Post Sign (Autodesk Fusion 360 design; units mm, degrees)
Autodesk Fusion 360 part; units mm, degrees
(part 1 of 5)
sketch "Sketch1" plane through (0, 0, 0) normal (0, 0, 1) x (1, 0, 0)
  spline S0 degree 3 poles (15.8654, 98.7935) (15.4934, 98.9562) (15.1331, 99.0376) (14.7843, 99.0376) knots 0 0 0 0 1 1 1 1
  spline S1 degree 3 poles (14.7843, 99.0376) (14.4356, 99.0376) (14.0868, 98.8167) (13.7381, 98.375) knots 0 0 0 0 1 1 1 1
  spline S2 degree 3 poles (13.7381, 98.375) (13.3894, 97.9332) (13.1568, 97.2939) (13.0406, 96.4569) knots 0 0 0 0 1 1 1 1
  line L0 (13.0406, 96.4569) -> (11.2969, 84.2509)
  spline S3 degree 3 poles (11.2969, 84.2509) (14.2263, 85.5296) (16.0979, 86.4829) (16.9117, 87.1106) knots 0 0 0 0 1 1 1 1
  line L1 (16.9117, 87.1106) -> (18.2369, 84.8089)
  spline S4 degree 3 poles (18.2369, 84.8089) (17.5394, 84.2742) (16.7024, 83.7975) (15.7259, 83.3791) knots 0 0 0 0 1 1 1 1
  spline S5 degree 3 poles (15.7259, 83.3791) (14.7495, 82.9606) (13.8078, 82.5653) (12.9011, 82.1933) knots 0 0 0 0 1 1 1 1
  spline S6 degree 3 poles (12.9011, 82.1933) (11.9944, 81.8446) (11.3202, 81.5772) (10.8784, 81.3912) knots 0 0 0 0 1 1 1 1
  line L2 (10.8784, 81.3912) -> (9.7276, 73.2307)
  spline S7 degree 3 poles (9.7276, 73.2307) (9.4253, 70.9987) (8.6232, 69.3596) (7.3212, 68.3134) knots 0 0 0 0 1 1 1 1
  spline S8 degree 3 poles (7.3212, 68.3134) (6.0425, 67.2439) (4.6243, 66.7092) (3.0666, 66.7092) knots 0 0 0 0 1 1 1 1
  spline S9 degree 3 poles (3.0666, 66.7092) (1.5321, 66.7092) (0.3115, 67.2788) (-0.5952, 68.418) knots 0 0 0 0 1 1 1 1
  spline S10 degree 3 poles (-0.5952, 68.418) (-1.5019, 69.534) (-1.9553, 70.7895) (-1.9553, 72.1844) knots 0 0 0 0 1 1 1 1
  spline S11 degree 3 poles (-1.9553, 72.1844) (-1.9553, 75.8346) (0.7184, 79.0779) (6.0658, 81.9143) knots 0 0 0 0 1 1 1 1
  line L3 (6.0658, 81.9143) -> (6.4145, 84.7391)
  spline S12 degree 3 poles (6.4145, 84.7391) (6.8563, 88.7381) (7.3096, 92.2138) (7.7746, 95.1665) knots 0 0 0 0 1 1 1 1
  spline S13 degree 3 poles (7.7746, 95.1665) (6.4494, 94.6318) (5.0544, 94.3644) (3.5897, 94.3644) knots 0 0 0 0 1 1 1 1
  spline S14 degree 3 poles (3.5897, 94.3644) (2.1482, 94.3644) (0.9741, 94.7597) (0.0674, 95.5502) knots 0 0 0 0 1 1 1 1
  spline S15 degree 3 poles (0.0674, 95.5502) (-0.8161, 96.3407) (-1.2578, 97.3752) (-1.2578, 98.654) knots 0 0 0 0 1 1 1 1
  spline S16 degree 3 poles (-1.2578, 98.654) (-1.2578, 99.9327) (-0.8044, 100.9324) (0.1023, 101.6531) knots 0 0 0 0 1 1 1 1
  spline S17 degree 3 poles (0.1023, 101.6531) (1.0323, 102.3971) (2.1947, 102.7691) (3.5897, 102.7691) knots 0 0 0 0 1 1 1 1
  spline S18 degree 3 poles (3.5897, 102.7691) (4.45, 102.7691) (5.6822, 102.5017) (7.2864, 101.967) knots 0 0 0 0 1 1 1 1
  spline S19 degree 3 poles (7.2864, 101.967) (8.9139, 101.4323) (10.1693, 101.1649) (11.0528, 101.1649) knots 0 0 0 0 1 1 1 1
  spline S20 degree 3 poles (11.0528, 101.1649) (12.6337, 101.1649) (13.959, 101.5718) (15.0284, 102.3855) knots 0 0 0 0 1 1 1 1
  spline S21 degree 3 poles (15.0284, 102.3855) (15.6097, 101.5718) (15.9003, 100.6069) (15.9003, 99.4909) knots 0 0 0 0 1 1 1 1
  spline S22 degree 3 poles (15.9003, 99.4909) (15.9003, 99.2584) (15.8887, 99.026) (15.8654, 98.7935) knots 0 0 0 0 1 1 1 1
  spline S23 degree 3 poles (2.1947, 97.7124) (2.1947, 97.3636) (2.3807, 97.0614) (2.7527, 96.8056) knots 0 0 0 0 1 1 1 1
  spline S24 degree 3 poles (2.7527, 96.8056) (3.1479, 96.5499) (3.7292, 96.422) (4.4964, 96.422) knots 0 0 0 0 1 1 1 1
  spline S25 degree 3 poles (4.4964, 96.422) (5.2869, 96.422) (6.3099, 96.7707) (7.5654, 97.4682) knots 0 0 0 0 1 1 1 1
  spline S26 degree 3 poles (7.5654, 97.4682) (6.6586, 97.6775) (5.7286, 97.91) (4.7754, 98.1657) knots 0 0 0 0 1 1 1 1
  spline S27 degree 3 poles (4.7754, 98.1657) (3.8222, 98.4447) (3.2526, 98.5842) (3.0666, 98.5842) knots 0 0 0 0 1 1 1 1
  spline S28 degree 3 poles (3.0666, 98.5842) (2.4854, 98.5842) (2.1947, 98.2936) (2.1947, 97.7124) knots 0 0 0 0 1 1 1 1
  spline S29 degree 3 poles (5.6822, 78.8803) (2.3575, 76.8808) (0.6951, 74.7651) (0.6951, 72.5332) knots 0 0 0 0 1 1 1 1
  spline S30 degree 3 poles (0.6951, 72.5332) (0.6951, 71.9054) (0.8579, 71.3707) (1.1834, 70.929) knots 0 0 0 0 1 1 1 1
  spline S31 degree 3 poles (1.1834, 70.929) (1.5554, 70.4175) (2.0204, 70.1617) (2.5784, 70.1617) knots 0 0 0 0 1 1 1 1
  spline S32 degree 3 poles (2.5784, 70.1617) (3.1596, 70.1617) (3.6595, 70.3361) (4.0779, 70.6848) knots 0 0 0 0 1 1 1 1
  spline S33 degree 3 poles (4.0779, 70.6848) (4.4964, 71.0336) (4.7522, 71.5916) (4.8452, 72.3588) knots 0 0 0 0 1 1 1 1
  line L4 (4.8452, 72.3588) -> (5.6822, 78.8803)
  spline S34 degree 3 poles (29.2909, 92.6905) (28.3377, 85.1576) (27.8611, 81.1471) (27.8611, 80.6589) knots 0 0 0 0 1 1 1 1
  spline S35 degree 3 poles (27.8611, 80.6589) (27.8611, 79.7289) (28.1982, 79.2639) (28.8724, 79.2639) knots 0 0 0 0 1 1 1 1
  spline S36 degree 3 poles (28.8724, 79.2639) (29.4769, 79.2639) (30.1279, 79.6708) (30.8254, 80.4845) knots 0 0 0 0 1 1 1 1
  spline S37 degree 3 poles (30.8254, 80.4845) (31.5461, 81.3215) (32.1157, 82.5653) (32.5342, 84.216) knots 0 0 0 0 1 1 1 1
  spline S38 degree 3 poles (32.5342, 84.216) (33.3014, 83.3791) (33.7664, 82.728) (33.9292, 82.2631) knots 0 0 0 0 1 1 1 1
  spline S39 degree 3 poles (33.9292, 82.2631) (33.3945, 80.0079) (32.5458, 78.4153) (31.3834, 77.4853) knots 0 0 0 0 1 1 1 1
  spline S40 degree 3 poles (31.3834, 77.4853) (30.2209, 76.5553) (29.0235, 76.0903) (27.7913, 76.0903) knots 0 0 0 0 1 1 1 1
  spline S41 degree 3 poles (27.7913, 76.0903) (25.7686, 76.0903) (24.4085, 76.8692) (23.711, 78.4269) knots 0 0 0 0 1 1 1 1
  spline S42 degree 3 poles (23.711, 78.4269) (22.502, 76.8692) (20.8862, 76.0903) (18.8635, 76.0903) knots 0 0 0 0 1 1 1 1
  spline S43 degree 3 poles (18.8635, 76.0903) (17.1896, 76.0903) (15.8992, 76.5088) (14.9925, 77.3458) knots 0 0 0 0 1 1 1 1
  spline S44 degree 3 poles (14.9925, 77.3458) (14.0857, 78.1828) (13.6324, 79.2755) (13.6324, 80.624) knots 0 0 0 0 1 1 1 1
  spline S45 degree 3 poles (13.6324, 80.624) (13.6324, 80.9495) (13.6905, 81.5191) (13.8068, 82.3328) knots 0 0 0 0 1 1 1 1
  spline S46 degree 3 poles (13.8068, 82.3328) (14.3415, 86.6572) (14.7484, 90.0982) (15.0274, 92.6556) knots 0 0 0 0 1 1 1 1
  spline S47 degree 3 poles (15.0274, 92.6556) (15.7481, 92.9113) (16.4107, 93.0392) (17.0152, 93.0392) knots 0 0 0 0 1 1 1 1
  spline S48 degree 3 poles (17.0152, 93.0392) (17.6197, 93.0392) (18.073, 93.0159) (18.3753, 92.9695) knots 0 0 0 0 1 1 1 1
  spline S49 degree 3 poles (18.3753, 92.9695) (18.6775, 92.923) (18.9681, 92.7486) (19.2471, 92.4463) knots 0 0 0 0 1 1 1 1
  spline S50 degree 3 poles (19.2471, 92.4463) (19.5261, 92.1441) (19.6656, 91.714) (19.6656, 91.156) knots 0 0 0 0 1 1 1 1
  line L5 (19.6656, 91.156) -> (18.5148, 82.2631)
  spline S51 degree 3 poles (18.5148, 82.2631) (18.4683, 81.9841) (18.445, 81.7284) (18.445, 81.4958) knots 0 0 0 0 1 1 1 1
  spline S52 degree 3 poles (18.445, 81.4958) (18.445, 80.1241) (19.0728, 79.4383) (20.3282, 79.4383) knots 0 0 0 0 1 1 1 1
  spline S53 degree 3 poles (20.3282, 79.4383) (21.4907, 79.4383) (22.4556, 80.0079) (23.2228, 81.1471) knots 0 0 0 0 1 1 1 1
  spline S54 degree 3 poles (23.2228, 81.1471) (23.2228, 81.4028) (23.2461, 81.8097) (23.2925, 82.3677) knots 0 0 0 0 1 1 1 1
  line L6 (23.2925, 82.3677) -> (24.4434, 91.6442)
  spline S55 degree 3 poles (24.4434, 91.6442) (24.6062, 92.0395) (24.9549, 92.365) (25.4896, 92.6207) knots 0 0 0 0 1 1 1 1
  spline S56 degree 3 poles (25.4896, 92.6207) (26.0243, 92.8997) (26.6869, 93.0392) (27.4774, 93.0392) knots 0 0 0 0 1 1 1 1
  spline S57 degree 3 poles (27.4774, 93.0392) (28.2912, 93.0392) (28.8957, 92.923) (29.2909, 92.6905) knots 0 0 0 0 1 1 1 1
  line L7 (40.9332, 80.2404) -> (41.7701, 87.9476)
  spline S58 degree 3 poles (41.7701, 87.9476) (41.7701, 88.5753) (41.6074, 89.0984) (41.2819, 89.5169) knots 0 0 0 0 1 1 1 1
  spline S59 degree 3 poles (41.2819, 89.5169) (40.9564, 89.9354) (40.4333, 90.1446) (39.7126, 90.1446) knots 0 0 0 0 1 1 1 1
  spline S60 degree 3 poles (39.7126, 90.1446) (38.9919, 90.1446) (38.3757, 89.854) (37.8642, 89.2728) knots 0 0 0 0 1 1 1 1
  spline S61 degree 3 poles (37.8642, 89.2728) (37.376, 88.7148) (37.0156, 87.9708) (36.7831, 87.0408) knots 0 0 0 0 1 1 1 1
  spline S62 degree 3 poles (36.7831, 87.0408) (36.6204, 85.7156) (36.3763, 83.7743) (36.0508, 81.2168) knots 0 0 0 0 1 1 1 1
  spline S63 degree 3 poles (36.0508, 81.2168) (35.7253, 78.6826) (35.5161, 77.0319) (35.423, 76.2647) knots 0 0 0 0 1 1 1 1
  line L8 (35.423, 76.2647) -> (30.7848, 76.2647)
  spline S64 degree 3 poles (30.7848, 76.2647) (32.4587, 90.5167) (33.4701, 99.2701) (33.8188, 102.525) knots 0 0 0 0 1 1 1 1
  spline S65 degree 3 poles (33.8188, 102.525) (34.3071, 102.711) (34.9697, 102.804) (35.8067, 102.804) knots 0 0 0 0 1 1 1 1
  spline S66 degree 3 poles (35.8067, 102.804) (37.6201, 102.804) (38.5268, 102.2693) (38.5268, 101.1998) knots 0 0 0 0 1 1 1 1
  line L9 (38.5268, 101.1998) -> (38.5268, 100.9905)
  spline S67 degree 3 poles (38.5268, 100.9905) (38.1316, 97.3403) (37.7131, 94.1319) (37.2714, 91.3652) knots 0 0 0 0 1 1 1 1
  spline S68 degree 3 poles (37.2714, 91.3652) (38.5036, 92.4812) (39.8986, 93.0392) (41.4563, 93.0392) knots 0 0 0 0 1 1 1 1
  spline S69 degree 3 poles (41.4563, 93.0392) (43.014, 93.0392) (44.2462, 92.644) (45.1529, 91.8535) knots 0 0 0 0 1 1 1 1
  spline S70 degree 3 poles (45.1529, 91.8535) (46.0597, 91.063) (46.513, 90.0633) (46.513, 88.8543) knots 0 0 0 0 1 1 1 1
  spline S71 degree 3 poles (46.513, 88.8543) (46.513, 88.5288) (46.4433, 87.9243) (46.3038, 87.0408) knots 0 0 0 0 1 1 1 1
  spline S72 degree 3 poles (46.3038, 87.0408) (45.7691, 83.5534) (45.5017, 81.5075) (45.5017, 80.903) knots 0 0 0 0 1 1 1 1
  spline S73 degree 3 poles (45.5017, 80.903) (45.5017, 79.8103) (45.8621, 79.2639) (46.5828, 79.2639) knots 0 0 0 0 1 1 1 1
  spline S74 degree 3 poles (46.5828, 79.2639) (47.1873, 79.2639) (47.8266, 79.6591) (48.5007, 80.4496) knots 0 0 0 0 1 1 1 1
  spline S75 degree 3 poles (48.5007, 80.4496) (49.1982, 81.2633) (49.7562, 82.5072) (50.1747, 84.1812) knots 0 0 0 0 1 1 1 1
  spline S76 degree 3 poles (50.1747, 84.1812) (50.9653, 83.3442) (51.4421, 82.6816) (51.6045, 82.1933) knots 0 0 0 0 1 1 1 1
  spline S77 degree 3 poles (51.6045, 82.1933) (50.3959, 78.1479) (48.2566, 76.1252) (45.1878, 76.1252) knots 0 0 0 0 1 1 1 1
  spline S78 degree 3 poles (45.1878, 76.1252) (43.7464, 76.1252) (42.6769, 76.567) (41.9794, 77.4504) knots 0 0 0 0 1 1 1 1
  spline S79 degree 3 poles (41.9794, 77.4504) (41.2819, 78.3339) (40.9332, 79.2639) (40.9332, 80.2404) knots 0 0 0 0 1 1 1 1
  spline S80 degree 3 poles (64.2664, 76.0903) (62.1276, 76.0903) (60.7092, 76.8343) (60.0117, 78.3223) knots 0 0 0 0 1 1 1 1
  spline S81 degree 3 poles (60.0117, 78.3223) (58.8031, 76.8111) (57.2452, 76.0555) (55.3386, 76.0555) knots 0 0 0 0 1 1 1 1
  spline S82 degree 3 poles (55.3386, 76.0555) (53.4553, 76.0555) (51.8631, 76.6948) (50.5608, 77.9735) knots 0 0 0 0 1 1 1 1
  spline S83 degree 3 poles (50.5608, 77.9735) (49.2824, 79.2523) (48.6427, 80.9379) (48.6427, 83.0303) knots 0 0 0 0 1 1 1 1
  spline S84 degree 3 poles (48.6427, 83.0303) (48.6427, 86.076) (49.538, 88.5056) (51.328, 90.319) knots 0 0 0 0 1 1 1 1
  spline S85 degree 3 poles (51.328, 90.319) (53.1186, 92.1325) (55.3854, 93.0392) (58.1285, 93.0392) knots 0 0 0 0 1 1 1 1
  spline S86 degree 3 poles (58.1285, 93.0392) (58.1982, 93.0392) (58.268, 93.0392) (58.3377, 93.0392) knots 0 0 0 0 1 1 1 1
  spline S87 degree 3 poles (58.3377, 93.0392) (59.5005, 93.0392) (60.5697, 92.8416) (61.5462, 92.4463) knots 0 0 0 0 1 1 1 1
  spline S88 degree 3 poles (61.5462, 92.4463) (62.1739, 92.8416) (62.9297, 93.0392) (63.813, 93.0392) knots 0 0 0 0 1 1 1 1
  spline S89 degree 3 poles (63.813, 93.0392) (64.7197, 93.0392) (65.3709, 92.923) (65.7659, 92.6905) knots 0 0 0 0 1 1 1 1
  spline S90 degree 3 poles (65.7659, 92.6905) (65.5567, 90.97) (65.336, 89.2728) (65.1033, 87.5988) knots 0 0 0 0 1 1 1 1
  spline S91 degree 3 poles (65.1033, 87.5988) (64.8712, 85.9481) (64.7083, 84.774) (64.6151, 84.0765) knots 0 0 0 0 1 1 1 1
  spline S92 degree 3 poles (64.6151, 84.0765) (64.4058, 82.4956) (64.3012, 81.3563) (64.3012, 80.6589) knots 0 0 0 0 1 1 1 1
  spline S93 degree 3 poles (64.3012, 80.6589) (64.3012, 79.7289) (64.6734, 79.2639) (65.4172, 79.2639) knots 0 0 0 0 1 1 1 1
  spline S94 degree 3 poles (65.4172, 79.2639) (65.9986, 79.2639) (66.6149, 79.6475) (67.2655, 80.4147) knots 0 0 0 0 1 1 1 1
  spline S95 degree 3 poles (67.2655, 80.4147) (67.9167, 81.2052) (68.4861, 82.4374) (68.9744, 84.1114) knots 0 0 0 0 1 1 1 1
  spline S96 degree 3 poles (68.9744, 84.1114) (69.6489, 83.5069) (70.1138, 82.8327) (70.3693, 82.0887) knots 0 0 0 0 1 1 1 1
  spline S97 degree 3 poles (70.3693, 82.0887) (69.6953, 79.88) (68.7885, 78.3223) (67.6492, 77.4156) knots 0 0 0 0 1 1 1 1
  spline S98 degree 3 poles (67.6492, 77.4156) (66.5103, 76.5321) (65.3823, 76.0903) (64.2664, 76.0903) knots 0 0 0 0 1 1 1 1
  spline S99 degree 3 poles (58.6516, 90.319) (57.164, 90.319) (55.9782, 89.7494) (55.0944, 88.6102) knots 0 0 0 0 1 1 1 1
  spline S100 degree 3 poles (55.0944, 88.6102) (54.2345, 87.4942) (53.7229, 85.8202) (53.56, 83.5883) knots 0 0 0 0 1 1 1 1
  spline S101 degree 3 poles (53.56, 83.5883) (53.5371, 83.3791) (53.5251, 83.1814) (53.5251, 82.9954) knots 0 0 0 0 1 1 1 1
  spline S102 degree 3 poles (53.5251, 82.9954) (53.5251, 81.8562) (53.7926, 80.9495) (54.3272, 80.2752) knots 0 0 0 0 1 1 1 1
  spline S103 degree 3 poles (54.3272, 80.2752) (54.8852, 79.601) (55.5946, 79.2639) (56.4545, 79.2639) knots 0 0 0 0 1 1 1 1
  spline S104 degree 3 poles (56.4545, 79.2639) (57.9192, 79.2639) (59.0238, 80.2985) (59.7676, 82.3677) knots 0 0 0 0 1 1 1 1
  line L10 (59.7676, 82.3677) -> (60.6046, 89.9005)
  spline S105 degree 3 poles (60.6046, 89.9005) (59.9305, 90.1795) (59.2793, 90.319) (58.6516, 90.319) knots 0 0 0 0 1 1 1 1
  spline S106 degree 3 poles (82.4308, 86.9362) (84.2677, 85.5877) (85.1859, 83.9952) (85.1859, 82.1585) knots 0 0 0 0 1 1 1 1
  spline S107 degree 3 poles (85.1859, 82.1585) (85.1859, 80.3217) (84.465, 78.8454) (83.0237, 77.7294) knots 0 0 0 0 1 1 1 1
  spline S108 degree 3 poles (83.0237, 77.7294) (81.5824, 76.6135) (79.7689, 76.0555) (77.5833, 76.0555) knots 0 0 0 0 1 1 1 1
  spline S109 degree 3 poles (77.5833, 76.0555) (76.1649, 76.0555) (74.9792, 76.4042) (74.0261, 77.1017) knots 0 0 0 0 1 1 1 1
  spline S110 degree 3 poles (74.0261, 77.1017) (73.096, 77.8224) (72.6312, 78.7059) (72.6312, 79.7521) knots 0 0 0 0 1 1 1 1
  spline S111 degree 3 poles (72.6312, 79.7521) (72.6312, 80.7984) (72.9799, 81.6237) (73.6774, 82.2282) knots 0 0 0 0 1 1 1 1
  spline S112 degree 3 poles (73.6774, 82.2282) (74.3749, 82.8559) (75.2468, 83.2396) (76.293, 83.3791) knots 0 0 0 0 1 1 1 1
  spline S113 degree 3 poles (76.293, 83.3791) (75.8047, 82.6816) (75.5606, 82.0073) (75.5606, 81.3563) knots 0 0 0 0 1 1 1 1
  spline S114 degree 3 poles (75.5606, 81.3563) (75.5606, 80.7286) (75.7813, 80.2171) (76.2232, 79.8219) knots 0 0 0 0 1 1 1 1
  spline S115 degree 3 poles (76.2232, 79.8219) (76.6651, 79.4267) (77.2231, 79.229) (77.8972, 79.229) knots 0 0 0 0 1 1 1 1
  spline S116 degree 3 poles (77.8972, 79.229) (78.5713, 79.229) (79.1292, 79.4731) (79.5712, 79.9614) knots 0 0 0 0 1 1 1 1
  spline S117 degree 3 poles (79.5712, 79.9614) (80.0131, 80.4729) (80.2338, 81.0541) (80.2338, 81.7051) knots 0 0 0 0 1 1 1 1
  spline S118 degree 3 poles (80.2338, 81.7051) (80.2338, 82.7746) (79.7341, 83.7278) (78.7342, 84.5648) knots 0 0 0 0 1 1 1 1
  spline S119 degree 3 poles (78.7342, 84.5648) (78.1298, 85.053) (77.4787, 85.5064) (76.7812, 85.9249) knots 0 0 0 0 1 1 1 1
  spline S120 degree 3 poles (76.7812, 85.9249) (76.0837, 86.3666) (75.7116, 86.5991) (75.6652, 86.6224) knots 0 0 0 0 1 1 1 1
  spline S121 degree 3 poles (75.6652, 86.6224) (75.5721, 86.6921) (75.4794, 86.7502) (75.3862, 86.7967) knots 0 0 0 0 1 1 1 1
  spline S122 degree 3 poles (75.3862, 86.7967) (74.9678, 86.3085) (74.3634, 85.6343) (73.5728, 84.774) knots 0 0 0 0 1 1 1 1
  spline S123 degree 3 poles (73.5728, 84.774) (72.7821, 83.937) (72.1544, 83.2628) (71.6896, 82.7513) knots 0 0 0 0 1 1 1 1
  spline S124 degree 3 poles (71.6896, 82.7513) (70.3878, 81.3331) (69.6554, 80.1474) (69.4925, 79.1941) knots 0 0 0 0 1 1 1 1
  spline S125 degree 3 poles (69.4925, 79.1941) (69.4462, 79.0082) (69.4228, 78.6478) (69.4228, 78.113) knots 0 0 0 0 1 1 1 1
  spline S126 degree 3 poles (69.4228, 78.113) (69.4228, 77.6015) (69.5737, 77.0668) (69.8761, 76.5088) knots 0 0 0 0 1 1 1 1
  spline S127 degree 3 poles (69.8761, 76.5088) (70.2015, 75.9508) (70.5851, 75.5324) (71.027, 75.2534) knots 0 0 0 0 1 1 1 1
  spline S128 degree 3 poles (71.027, 75.2534) (71.4689, 74.9744) (71.8988, 74.7535) (72.3173, 74.5907) knots 0 0 0 0 1 1 1 1
  spline S129 degree 3 poles (72.3173, 74.5907) (72.7592, 74.4048) (73.1309, 74.2769) (73.4333, 74.2071) knots 0 0 0 0 1 1 1 1
  spline S130 degree 3 poles (73.4333, 74.2071) (73.7586, 74.1374) (73.9215, 74.0909) (73.9215, 74.0676) knots 0 0 0 0 1 1 1 1
  spline S131 degree 3 poles (73.9215, 74.0676) (73.9215, 73.9049) (73.666, 73.7189) (73.1543, 73.5096) knots 0 0 0 0 1 1 1 1
  spline S132 degree 3 poles (73.1543, 73.5096) (72.2012, 73.1609) (71.2013, 72.9865) (70.1551, 72.9865) knots 0 0 0 0 1 1 1 1
  spline S133 degree 3 poles (70.1551, 72.9865) (69.1323, 72.9865) (68.1324, 73.3585) (67.1559, 74.1025) knots 0 0 0 0 1 1 1 1
  spline S134 degree 3 poles (67.1559, 74.1025) (65.8307, 75.1255) (65.1681, 76.4856) (65.1681, 78.1828) knots 0 0 0 0 1 1 1 1
  spline S135 degree 3 poles (65.1681, 78.1828) (65.1681, 79.229) (65.4356, 80.2636) (65.9702, 81.2866) knots 0 0 0 0 1 1 1 1
  spline S136 degree 3 poles (65.9702, 81.2866) (66.9233, 83.1001) (69.1552, 85.5877) (72.6661, 88.7497) knots 0 0 0 0 1 1 1 1
  spline S137 degree 3 poles (72.6661, 88.7497) (71.8057, 89.6099) (71.3757, 90.5283) (71.3757, 91.5047) knots 0 0 0 0 1 1 1 1
  spline S138 degree 3 poles (71.3757, 91.5047) (71.3757, 92.4812) (71.7359, 93.3066) (72.4568, 93.9808) knots 0 0 0 0 1 1 1 1
  spline S139 degree 3 poles (72.4568, 93.9808) (73.2006, 94.655) (74.0725, 94.9922) (75.0724, 94.9922) knots 0 0 0 0 1 1 1 1
  spline S140 degree 3 poles (75.0724, 94.9922) (75.9791, 94.9922) (76.7698, 94.6318) (77.4438, 93.9111) knots 0 0 0 0 1 1 1 1
  spline S141 degree 3 poles (77.4438, 93.9111) (77.8857, 93.4228) (78.1064, 92.8067) (78.1064, 92.0627) knots 0 0 0 0 1 1 1 1
  spline S142 degree 3 poles (78.1064, 92.0627) (78.1064, 91.3188) (77.8623, 90.4818) (77.3741, 89.5518) knots 0 0 0 0 1 1 1 1
  spline S143 degree 3 poles (77.3741, 89.5518) (79.8616, 88.4358) (81.5475, 87.564) (82.4308, 86.9362) knots 0 0 0 0 1 1 1 1
  spline S144 degree 3 poles (74.8631, 90.877) (75.4211, 91.4583) (75.7001, 91.8768) (75.7001, 92.1325) knots 0 0 0 0 1 1 1 1
  spline S145 degree 3 poles (75.7001, 92.1325) (75.7001, 92.7137) (75.4445, 93.0276) (74.9329, 93.0741) knots 0 0 0 0 1 1 1 1
  spline S146 degree 3 poles (74.9329, 93.0741) (74.3515, 93.0741) (74.061, 92.7486) (74.061, 92.0976) knots 0 0 0 0 1 1 1 1
  spline S147 degree 3 poles (74.061, 92.0976) (74.061, 91.7024) (74.3286, 91.2955) (74.8631, 90.877) knots 0 0 0 0 1 1 1 1
  line L11 (95.4962, 75.9508) -> (85.8012, 76.1601)
  spline S148 degree 3 poles (85.8012, 76.1601) (85.4993, 76.1601) (85.3478, 76.567) (85.3478, 77.3807) knots 0 0 0 0 1 1 1 1
  spline S149 degree 3 poles (85.3478, 77.3807) (85.3478, 78.2177) (85.5222, 78.8687) (85.8709, 79.3336) knots 0 0 0 0 1 1 1 1
  spline S150 degree 3 poles (85.8709, 79.3336) (86.2197, 80.2636) (87.1847, 81.6237) (88.7655, 83.4139) knots 0 0 0 0 1 1 1 1
  spline S151 degree 3 poles (88.7655, 83.4139) (89.2771, 83.9952) (90.2302, 85.0414) (91.6252, 86.5526) knots 0 0 0 0 1 1 1 1
  spline S152 degree 3 poles (91.6252, 86.5526) (93.0201, 88.0638) (93.9388, 89.0984) (94.3802, 89.6564) knots 0 0 0 0 1 1 1 1
  line L12 (94.3802, 89.6564) -> (92.5319, 89.761)
  spline S153 degree 3 poles (92.5319, 89.761) (92.1832, 88.9241) (91.672, 88.2382) (90.9974, 87.7035) knots 0 0 0 0 1 1 1 1
  spline S154 degree 3 poles (90.9974, 87.7035) (90.3468, 87.1919) (89.6144, 86.9362) (88.8004, 86.9362) knots 0 0 0 0 1 1 1 1
  spline S155 degree 3 poles (88.8004, 86.9362) (87.8707, 86.9362) (87.1149, 87.2036) (86.5335, 87.7383) knots 0 0 0 0 1 1 1 1
  spline S156 degree 3 poles (86.5335, 87.7383) (85.9526, 88.2963) (85.6617, 89.0635) (85.6617, 90.04) knots 0 0 0 0 1 1 1 1
  spline S157 degree 3 poles (85.6617, 90.04) (85.6617, 91.0165) (85.999, 91.7953) (86.673, 92.3766) knots 0 0 0 0 1 1 1 1
  spline S158 degree 3 poles (86.673, 92.3766) (87.3476, 92.9579) (88.2773, 93.2485) (89.463, 93.2485) knots 0 0 0 0 1 1 1 1
  line L13 (89.463, 93.2485) -> (99.158, 93.0392)
  spline S159 degree 3 poles (99.158, 93.0392) (99.4604, 93.0392) (99.6114, 92.644) (99.6114, 91.8535) knots 0 0 0 0 1 1 1 1
  spline S160 degree 3 poles (99.6114, 91.8535) (99.6114, 91.0398) (99.4604, 90.412) (99.158, 89.9703) knots 0 0 0 0 1 1 1 1
  spline S161 degree 3 poles (99.158, 89.9703) (98.879, 89.4588) (98.4725, 88.9124) (97.9374, 88.3312) knots 0 0 0 0 1 1 1 1
  spline S162 degree 3 poles (97.9374, 88.3312) (97.4263, 87.7732) (96.6705, 87.0176) (95.6706, 86.0644) knots 0 0 0 0 1 1 1 1
  spline S163 degree 3 poles (95.6706, 86.0644) (94.6712, 85.1344) (93.9737, 84.4718) (93.5781, 84.0765) knots 0 0 0 0 1 1 1 1
  spline S164 degree 3 poles (93.5781, 84.0765) (92.0207, 82.5188) (90.8579, 81.0192) (90.0907, 79.5778) knots 0 0 0 0 1 1 1 1
  line L14 (90.0907, 79.5778) -> (92.4273, 79.4383)
  spline S165 degree 3 poles (92.4273, 79.4383) (92.776, 80.2752) (93.2762, 80.9495) (93.9269, 81.461) knots 0 0 0 0 1 1 1 1
  spline S166 degree 3 poles (93.9269, 81.461) (94.6014, 81.9957) (95.3453, 82.2631) (96.1588, 82.2631) knots 0 0 0 0 1 1 1 1
  spline S167 degree 3 poles (96.1588, 82.2631) (97.089, 82.2631) (97.8447, 81.9841) (98.4256, 81.4261) knots 0 0 0 0 1 1 1 1
  spline S168 degree 3 poles (98.4256, 81.4261) (99.0071, 80.8914) (99.2975, 80.1357) (99.2975, 79.1593) knots 0 0 0 0 1 1 1 1
  spline S169 degree 3 poles (99.2975, 79.1593) (99.2975, 78.1828) (98.9607, 77.404) (98.2862, 76.8227) knots 0 0 0 0 1 1 1 1
  spline S170 degree 3 poles (98.2862, 76.8227) (97.6121, 76.2414) (96.6819, 75.9508) (95.4962, 75.9508) knots 0 0 0 0 1 1 1 1
  spline S171 degree 3 poles (89.184, 90.0052) (88.3704, 90.0052) (87.9634, 89.7378) (87.9634, 89.203) knots 0 0 0 0 1 1 1 1
  spline S172 degree 3 poles (87.9634, 89.203) (87.9634, 88.6683) (88.2658, 88.4009) (88.8701, 88.4009) knots 0 0 0 0 1 1 1 1
  spline S173 degree 3 poles (88.8701, 88.4009) (89.7768, 88.4009) (90.4977, 88.8892) (91.0323, 89.8657) knots 0 0 0 0 1 1 1 1
  line L15 (91.0323, 89.8657) -> (89.6025, 89.9703)
  spline S174 degree 3 poles (89.6025, 89.9703) (89.463, 89.9935) (89.3235, 90.0052) (89.184, 90.0052) knots 0 0 0 0 1 1 1 1
  spline S175 degree 3 poles (95.7752, 79.1941) (96.5893, 79.1941) (96.9958, 79.4615) (96.9958, 79.9963) knots 0 0 0 0 1 1 1 1
  spline S176 degree 3 poles (96.9958, 79.9963) (96.9958, 80.531) (96.6939, 80.7984) (96.0891, 80.7984) knots 0 0 0 0 1 1 1 1
  spline S177 degree 3 poles (96.0891, 80.7984) (95.1823, 80.7984) (94.4619, 80.3101) (93.9269, 79.3336) knots 0 0 0 0 1 1 1 1
  line L16 (93.9269, 79.3336) -> (95.3567, 79.229)
  spline S178 degree 3 poles (95.3567, 79.229) (95.4962, 79.2058) (95.6357, 79.1941) (95.7752, 79.1941) knots 0 0 0 0 1 1 1 1
  line L17 (0.6979, -154.6893) -> (-1.247, -154.6893)
  line L18 (-1.247, -154.6893) -> (-1.247, -153.5509)
  line L19 (-1.247, -153.5509) -> (0.6979, -153.5509)
  spline S179 degree 3 poles (0.6979, -153.5509) (1.2566, -153.5509) (1.7257, -153.3402) (2.1052, -152.9187) knots 0 0 0 0 1 1 1 1
  spline S180 degree 3 poles (2.1052, -152.9187) (2.4847, -152.4967) (2.6744, -151.9382) (2.6744, -151.2422) knots 0 0 0 0 1 1 1 1
  line L20 (2.6744, -151.2422) -> (2.6744, -134.1967)
  line L21 (2.6744, -134.1967) -> (3.8128, -134.1967)
  line L22 (3.8128, -134.1967) -> (3.8128, -151.2422)
  spline S181 degree 3 poles (3.8128, -151.2422) (3.8128, -152.2436) (3.5124, -153.0711) (2.9116, -153.7248) knots 0 0 0 0 1 1 1 1
  spline S182 degree 3 poles (2.9116, -153.7248) (2.3107, -154.3679) (1.5728, -154.6893) (0.6979, -154.6893) knots 0 0 0 0 1 1 1 1
  line L23 (0.6979, -156.9666) -> (-1.247, -156.9666)
  line L24 (-1.247, -156.9666) -> (-1.247, -155.8277)
  line L25 (-1.247, -155.8277) -> (0.6979, -155.8277)
  spline S183 degree 3 poles (0.6979, -155.8277) (1.8785, -155.8277) (2.88, -155.3798) (3.7022, -154.484) knots 0 0 0 0 1 1 1 1
  spline S184 degree 3 poles (3.7022, -154.484) (4.5349, -153.5877) (4.9513, -152.5071) (4.9513, -151.2422) knots 0 0 0 0 1 1 1 1
  line L26 (4.9513, -151.2422) -> (4.9513, -134.1967)
  line L27 (4.9513, -134.1967) -> (6.0898, -134.1967)
  line L28 (6.0898, -134.1967) -> (6.0898, -151.2422)
  spline S185 degree 3 poles (6.0898, -151.2422) (6.0898, -152.8235) (5.5627, -154.1726) (4.5086, -155.2901) knots 0 0 0 0 1 1 1 1
  spline S186 degree 3 poles (4.5086, -155.2901) (3.465, -156.4076) (2.1948, -156.9666) (0.6979, -156.9666) knots 0 0 0 0 1 1 1 1
  line L29 (0.6979, -159.2434) -> (-1.247, -159.2434)
  line L30 (-1.247, -159.2434) -> (-1.247, -158.105)
  line L31 (-1.247, -158.105) -> (0.6979, -158.105)
  spline S187 degree 3 poles (0.6979, -158.105) (2.511, -158.105) (4.05, -157.4354) (5.315, -156.0967) knots 0 0 0 0 1 1 1 1
  spline S188 degree 3 poles (5.315, -156.0967) (6.5905, -154.758) (7.2283, -153.1399) (7.2283, -151.2422) knots 0 0 0 0 1 1 1 1
  line L32 (7.2283, -151.2422) -> (7.2283, -134.1967)
  line L33 (7.2283, -134.1967) -> (8.3668, -134.1967)
  line L34 (8.3668, -134.1967) -> (8.3668, -151.2422)
  spline S189 degree 3 poles (8.3668, -151.2422) (8.3668, -152.6865) (8.0242, -154.0252) (7.339, -155.2587) knots 0 0 0 0 1 1 1 1
  spline S190 degree 3 poles (7.339, -155.2587) (6.6643, -156.4813) (5.7367, -157.4513) (4.556, -158.1682) knots 0 0 0 0 1 1 1 1
  spline S191 degree 3 poles (4.556, -158.1682) (3.3754, -158.8846) (2.0894, -159.2434) (0.6979, -159.2434) knots 0 0 0 0 1 1 1 1
  line L35 (0.6979, -161.5201) -> (-1.247, -161.5201)
  line L36 (-1.247, -161.5201) -> (-1.247, -160.3817)
  line L37 (-1.247, -160.3817) -> (0.6979, -160.3817)
  spline S192 degree 3 poles (0.6979, -160.3817) (1.8996, -160.3817) (3.0434, -160.1391) (4.1291, -159.6544) knots 0 0 0 0 1 1 1 1
  spline S193 degree 3 poles (4.1291, -159.6544) (5.2149, -159.1696) (6.1478, -158.521) (6.9279, -157.7094) knots 0 0 0 0 1 1 1 1
  spline S194 degree 3 poles (6.9279, -157.7094) (7.7185, -156.8874) (8.3457, -155.9124) (8.8095, -154.7844) knots 0 0 0 0 1 1 1 1
  spline S195 degree 3 poles (8.8095, -154.7844) (9.2733, -153.6565) (9.5052, -152.4758) (9.5052, -151.2422) knots 0 0 0 0 1 1 1 1
  line L38 (9.5052, -151.2422) -> (9.5052, -134.1967)
  line L39 (9.5052, -134.1967) -> (10.6437, -134.1967)
  line L40 (10.6437, -134.1967) -> (10.6437, -151.2422)
  spline S196 degree 3 poles (10.6437, -151.2422) (10.6437, -152.6337) (10.3802, -153.9619) (9.8531, -155.2268) knots 0 0 0 0 1 1 1 1
  spline S197 degree 3 poles (9.8531, -155.2268) (9.3366, -156.4918) (8.6303, -157.5883) (7.7343, -158.516) knots 0 0 0 0 1 1 1 1
  spline S198 degree 3 poles (7.7343, -158.516) (6.8488, -159.4332) (5.7894, -160.1606) (4.556, -160.6981) knots 0 0 0 0 1 1 1 1
  spline S199 degree 3 poles (4.556, -160.6981) (3.3332, -161.2461) (2.0472, -161.5201) (0.6979, -161.5201) knots 0 0 0 0 1 1 1 1
  line L41 (28.4956, -150.2936) -> (28.4956, -137.6124)
  line L42 (28.4956, -137.6124) -> (29.6341, -137.6124)
  line L43 (29.6341, -137.6124) -> (29.6341, -150.2936)
  spline S200 degree 3 poles (29.6341, -150.2936) (29.6341, -151.4953) (29.1702, -152.5286) (28.2426, -153.3929) knots 0 0 0 0 1 1 1 1
  spline S201 degree 3 poles (28.2426, -153.3929) (27.3255, -154.2573) (26.2186, -154.6893) (24.9221, -154.6893) knots 0 0 0 0 1 1 1 1
  spline S202 degree 3 poles (24.9221, -154.6893) (23.6254, -154.6893) (22.5133, -154.2573) (21.5857, -153.3929) knots 0 0 0 0 1 1 1 1
  spline S203 degree 3 poles (21.5857, -153.3929) (20.6686, -152.5286) (20.21, -151.4953) (20.21, -150.2936) knots 0 0 0 0 1 1 1 1
  line L44 (20.21, -150.2936) -> (20.21, -137.6124)
  line L45 (20.21, -137.6124) -> (21.3485, -137.6124)
  line L46 (21.3485, -137.6124) -> (21.3485, -150.2936)
  spline S204 degree 3 poles (21.3485, -150.2936) (21.3485, -151.1894) (21.6963, -151.9591) (22.3921, -152.6023) knots 0 0 0 0 1 1 1 1
  spline S205 degree 3 poles (22.3921, -152.6023) (23.0984, -153.2345) (23.9417, -153.5509) (24.9221, -153.5509) knots 0 0 0 0 1 1 1 1
  spline S206 degree 3 poles (24.9221, -153.5509) (25.9024, -153.5509) (26.7405, -153.2345) (27.4361, -152.6023) knots 0 0 0 0 1 1 1 1
  spline S207 degree 3 poles (27.4361, -152.6023) (28.1424, -151.9591) (28.4956, -151.1894) (28.4956, -150.2936) knots 0 0 0 0 1 1 1 1
  line L47 (30.7725, -150.2936) -> (30.7725, -137.6124)
  line L48 (30.7725, -137.6124) -> (31.911, -137.6124)
  line L49 (31.911, -137.6124) -> (31.911, -150.2936)
  spline S208 degree 3 poles (31.911, -150.2936) (31.911, -152.1385) (31.2258, -153.7143) (29.8554, -155.0216) knots 0 0 0 0 1 1 1 1
  spline S209 degree 3 poles (29.8554, -155.0216) (28.485, -156.3179) (26.8406, -156.9666) (24.9221, -156.9666) knots 0 0 0 0 1 1 1 1
  spline S210 degree 3 poles (24.9221, -156.9666) (23.0035, -156.9666) (21.3591, -156.3179) (19.9887, -155.0216) knots 0 0 0 0 1 1 1 1
  spline S211 degree 3 poles (19.9887, -155.0216) (18.6183, -153.7143) (17.9331, -152.1385) (17.9331, -150.2936) knots 0 0 0 0 1 1 1 1
  line L50 (17.9331, -150.2936) -> (17.9331, -137.6124)
  line L51 (17.9331, -137.6124) -> (19.0716, -137.6124)
  line L52 (19.0716, -137.6124) -> (19.0716, -150.2936)
  spline S212 degree 3 poles (19.0716, -150.2936) (19.0716, -151.8221) (19.6408, -153.1294) (20.7793, -154.215) knots 0 0 0 0 1 1 1 1
  spline S213 degree 3 poles (20.7793, -154.215) (21.9283, -155.2901) (23.3092, -155.8277) (24.9221, -155.8277) knots 0 0 0 0 1 1 1 1
  spline S214 degree 3 poles (24.9221, -155.8277) (26.5243, -155.8277) (27.9, -155.2901) (29.049, -154.215) knots 0 0 0 0 1 1 1 1
  spline S215 degree 3 poles (29.049, -154.215) (30.198, -153.1294) (30.7725, -151.8221) (30.7725, -150.2936) knots 0 0 0 0 1 1 1 1
  line L53 (33.0494, -150.2936) -> (33.0494, -137.6124)
  line L54 (33.0494, -137.6124) -> (34.1879, -137.6124)
  line L55 (34.1879, -137.6124) -> (34.1879, -150.2936)
  spline S216 degree 3 poles (34.1879, -150.2936) (34.1879, -151.9063) (33.7715, -153.4034) (32.9388, -154.7844) knots 0 0 0 0 1 1 1 1
  spline S217 degree 3 poles (32.9388, -154.7844) (32.106, -156.1545) (30.9781, -157.2406) (29.555, -158.0417) knots 0 0 0 0 1 1 1 1
  spline S218 degree 3 poles (29.555, -158.0417) (28.1319, -158.8428) (26.5876, -159.2434) (24.9221, -159.2434) knots 0 0 0 0 1 1 1 1
  spline S219 degree 3 poles (24.9221, -159.2434) (23.2565, -159.2434) (21.7122, -158.8428) (20.2891, -158.0417) knots 0 0 0 0 1 1 1 1
  spline S220 degree 3 poles (20.2891, -158.0417) (18.866, -157.2406) (17.7381, -156.1545) (16.9053, -154.7844) knots 0 0 0 0 1 1 1 1
  spline S221 degree 3 poles (16.9053, -154.7844) (16.0725, -153.4034) (15.6561, -151.9063) (15.6561, -150.2936) knots 0 0 0 0 1 1 1 1
  line L56 (15.6561, -150.2936) -> (15.6561, -137.6124)
  line L57 (15.6561, -137.6124) -> (16.7946, -137.6124)
  line L58 (16.7946, -137.6124) -> (16.7946, -150.2936)
  spline S222 degree 3 poles (16.7946, -150.2936) (16.7946, -151.6956) (17.1583, -152.9974) (17.8856, -154.1991) knots 0 0 0 0 1 1 1 1
  spline S223 degree 3 poles (17.8856, -154.1991) (18.613, -155.4007) (19.5986, -156.3548) (20.8425, -157.0612) knots 0 0 0 0 1 1 1 1
  spline S224 degree 3 poles (20.8425, -157.0612) (22.097, -157.7567) (23.4568, -158.105) (24.9221, -158.105) knots 0 0 0 0 1 1 1 1
  spline S225 degree 3 poles (24.9221, -158.105) (26.3873, -158.105) (27.7418, -157.7567) (28.9858, -157.0612) knots 0 0 0 0 1 1 1 1
  spline S226 degree 3 poles (28.9858, -157.0612) (30.2402, -156.3548) (31.2311, -155.4007) (31.9584, -154.1991) knots 0 0 0 0 1 1 1 1
  spline S227 degree 3 poles (31.9584, -154.1991) (32.6858, -152.9974) (33.0494, -151.6956) (33.0494, -150.2936) knots 0 0 0 0 1 1 1 1
  line L59 (35.3264, -150.2936) -> (35.3264, -137.6124)
  line L60 (35.3264, -137.6124) -> (36.4649, -137.6124)
  line L61 (36.4649, -137.6124) -> (36.4649, -150.2936)
  spline S228 degree 3 poles (36.4649, -150.2936) (36.4649, -151.8116) (36.1592, -153.2664) (35.5478, -154.6579) knots 0 0 0 0 1 1 1 1
  spline S229 degree 3 poles (35.5478, -154.6579) (34.9364, -156.0389) (34.1142, -157.2301) (33.0811, -158.2315) knots 0 0 0 0 1 1 1 1
  spline S230 degree 3 poles (33.0811, -158.2315) (32.048, -159.2329) (30.8199, -160.0285) (29.3969, -160.6189) knots 0 0 0 0 1 1 1 1
  spline S231 degree 3 poles (29.3969, -160.6189) (27.9738, -161.2197) (26.4822, -161.5201) (24.9221, -161.5201) knots 0 0 0 0 1 1 1 1
  spline S232 degree 3 poles (24.9221, -161.5201) (23.3619, -161.5201) (21.8703, -161.2197) (20.4472, -160.6189) knots 0 0 0 0 1 1 1 1
  spline S233 degree 3 poles (20.4472, -160.6189) (19.0241, -160.0285) (17.7961, -159.2329) (16.763, -158.2315) knots 0 0 0 0 1 1 1 1
  spline S234 degree 3 poles (16.763, -158.2315) (15.7299, -157.2301) (14.9077, -156.0389) (14.2963, -154.6579) knots 0 0 0 0 1 1 1 1
  spline S235 degree 3 poles (14.2963, -154.6579) (13.6849, -153.2664) (13.3792, -151.8116) (13.3792, -150.2936) knots 0 0 0 0 1 1 1 1
  line L62 (13.3792, -150.2936) -> (13.3792, -137.6124)
  line L63 (13.3792, -137.6124) -> (14.5177, -137.6124)
  line L64 (14.5177, -137.6124) -> (14.5177, -150.2936)
  spline S236 degree 3 poles (14.5177, -150.2936) (14.5177, -152.1066) (14.9815, -153.788) (15.9091, -155.3374) knots 0 0 0 0 1 1 1 1
  spline S237 degree 3 poles (15.9091, -155.3374) (16.8473, -156.8874) (18.1123, -158.1154) (19.704, -159.0221) knots 0 0 0 0 1 1 1 1
  spline S238 degree 3 poles (19.704, -159.0221) (21.3064, -159.9284) (23.0457, -160.3817) (24.9221, -160.3817) knots 0 0 0 0 1 1 1 1
  spline S239 degree 3 poles (24.9221, -160.3817) (26.7984, -160.3817) (28.5325, -159.9284) (30.1242, -159.0221) knots 0 0 0 0 1 1 1 1
  spline S240 degree 3 poles (30.1242, -159.0221) (31.7265, -158.1154) (32.9915, -156.8874) (33.9191, -155.3374) knots 0 0 0 0 1 1 1 1
  spline S241 degree 3 poles (33.9191, -155.3374) (34.8573, -153.788) (35.3264, -152.1066) (35.3264, -150.2936) knots 0 0 0 0 1 1 1 1
  line L65 (62.1121, -137.6124) -> (63.2505, -137.6124)
  line L66 (63.2505, -137.6124) -> (63.2505, -160.3817)
  line L67 (63.2505, -160.3817) -> (62.1121, -160.3817)
  line L68 (62.1121, -160.3817) -> (62.1121, -137.6124)
  line L69 (39.3269, -137.6124) -> (40.4654, -137.6124)
  line L70 (40.4654, -137.6124) -> (40.4654, -160.3817)
  line L71 (40.4654, -160.3817) -> (39.3269, -160.3817)
  line L72 (39.3269, -160.3817) -> (39.3269, -137.6124)
  line L73 (59.8353, -137.6124) -> (60.9737, -137.6124)
  line L74 (60.9737, -137.6124) -> (60.9737, -160.3817)
  line L75 (60.9737, -160.3817) -> (59.8353, -160.3817)
  line L76 (59.8353, -160.3817) -> (59.8353, -137.6124)
  line L77 (57.5581, -137.6124) -> (58.6969, -137.6124)
  line L78 (58.6969, -137.6124) -> (58.6969, -160.3817)
  line L79 (58.6969, -160.3817) -> (57.5581, -160.3817)
  line L80 (57.5581, -160.3817) -> (57.5581, -137.6124)
  line L81 (55.2813, -137.6124) -> (56.4197, -137.6124)
  line L82 (56.4197, -137.6124) -> (56.4197, -160.3817)
  line L83 (56.4197, -160.3817) -> (55.2813, -160.3817)
  line L84 (55.2813, -160.3817) -> (55.2813, -151.2741)
  line L85 (55.2813, -151.2741) -> (47.2962, -151.2741)
  line L86 (47.2962, -151.2741) -> (47.2962, -160.3817)
  line L87 (47.2962, -160.3817) -> (46.1577, -160.3817)
  line L88 (46.1577, -160.3817) -> (46.1577, -137.6124)
  line L89 (46.1577, -137.6124) -> (47.2962, -137.6124)
  line L90 (47.2962, -137.6124) -> (47.2962, -145.5816)
  line L91 (47.2962, -145.5816) -> (55.2813, -145.5816)
  line L92 (55.2813, -145.5816) -> (55.2813, -137.6124)
  line L93 (43.8808, -137.6124) -> (45.0192, -137.6124)
  line L94 (45.0192, -137.6124) -> (45.0192, -160.3817)
  line L95 (45.0192, -160.3817) -> (43.8808, -160.3817)
  line L96 (43.8808, -160.3817) -> (43.8808, -137.6124)
  line L97 (41.6038, -137.6124) -> (42.7423, -137.6124)
  line L98 (42.7423, -137.6124) -> (42.7423, -160.3817)
  line L99 (42.7423, -160.3817) -> (41.6038, -160.3817)
  line L100 (41.6038, -160.3817) -> (41.6038, -137.6124)
  line L101 (55.2813, -150.1357) -> (55.2813, -148.9968)
  line L102 (55.2813, -148.9968) -> (47.2962, -148.9968)
  line L103 (47.2962, -148.9968) -> (47.2962, -150.1357)
  line L104 (47.2962, -150.1357) -> (55.2813, -150.1357)
  line L105 (55.2813, -147.8584) -> (55.2813, -146.72)
  line L106 (55.2813, -146.72) -> (47.2962, -146.72)
  line L107 (47.2962, -146.72) -> (47.2962, -147.8584)
  line L108 (47.2962, -147.8584) -> (55.2813, -147.8584)
  spline S242 degree 3 poles (82.3989, -149.1552) (82.3989, -147.8056) (81.9825, -146.7624) (81.15, -146.0245) knots 0 0 0 0 1 1 1 1
  spline S243 degree 3 poles (81.15, -146.0245) (80.317, -145.2867) (79.2154, -144.9175) (77.8454, -144.9175) knots 0 0 0 0 1 1 1 1
  spline S244 degree 3 poles (77.8454, -144.9175) (76.6856, -144.9175) (75.6897, -145.3181) (74.8567, -146.1192) knots 0 0 0 0 1 1 1 1
  spline S245 degree 3 poles (74.8567, -146.1192) (74.0237, -146.9203) (73.6077, -147.8798) (73.6077, -148.9968) knots 0 0 0 0 1 1 1 1
  spline S246 degree 3 poles (73.6077, -148.9968) (73.6077, -149.6295) (73.6919, -150.199) (73.8607, -150.7046) knots 0 0 0 0 1 1 1 1
  spline S247 degree 3 poles (73.8607, -150.7046) (74.0291, -151.2004) (74.2558, -151.6164) (74.5403, -151.9536) knots 0 0 0 0 1 1 1 1
  spline S248 degree 3 poles (74.5403, -151.9536) (74.8357, -152.2805) (75.1835, -152.555) (75.584, -152.7762) knots 0 0 0 0 1 1 1 1
  spline S249 degree 3 poles (75.584, -152.7762) (75.9846, -152.9869) (76.4011, -153.1399) (76.833, -153.2345) knots 0 0 0 0 1 1 1 1
  spline S250 degree 3 poles (76.833, -153.2345) (77.2759, -153.3297) (77.7452, -153.377) (78.2404, -153.377) knots 0 0 0 0 1 1 1 1
  spline S251 degree 3 poles (78.2404, -153.377) (79.4421, -153.377) (80.5387, -153.0816) (81.5296, -152.4917) knots 0 0 0 0 1 1 1 1
  line L109 (81.5296, -152.4917) -> (81.5296, -153.6301)
  spline S252 degree 3 poles (81.5296, -153.6301) (80.5068, -154.1676) (79.4053, -154.4362) (78.2245, -154.4362) knots 0 0 0 0 1 1 1 1
  spline S253 degree 3 poles (78.2245, -154.4362) (77.4657, -154.4362) (76.7488, -154.336) (76.0743, -154.1358) knots 0 0 0 0 1 1 1 1
  spline S254 degree 3 poles (76.0743, -154.1358) (75.4102, -153.925) (74.8038, -153.6142) (74.2558, -153.2031) knots 0 0 0 0 1 1 1 1
  spline S255 degree 3 poles (74.2558, -153.2031) (73.7078, -152.7812) (73.2704, -152.2122) (72.9436, -151.4953) knots 0 0 0 0 1 1 1 1
  spline S256 degree 3 poles (72.9436, -151.4953) (72.6272, -150.7679) (72.4693, -149.9354) (72.4693, -148.9968) knots 0 0 0 0 1 1 1 1
  spline S257 degree 3 poles (72.4693, -148.9968) (72.4693, -147.5426) (72.9804, -146.309) (74.0027, -145.2971) knots 0 0 0 0 1 1 1 1
  spline S258 degree 3 poles (74.0027, -145.2971) (75.0256, -144.2848) (76.3059, -143.7791) (77.8454, -143.7791) knots 0 0 0 0 1 1 1 1
  spline S259 degree 3 poles (77.8454, -143.7791) (79.5423, -143.7791) (80.9128, -144.2589) (81.9565, -145.2179) knots 0 0 0 0 1 1 1 1
  spline S260 degree 3 poles (81.9565, -145.2179) (83.0102, -146.1665) (83.5373, -147.4793) (83.5373, -149.1552) knots 0 0 0 0 1 1 1 1
  line L110 (83.5373, -149.1552) -> (83.5373, -160.3817)
  line L111 (83.5373, -160.3817) -> (82.3989, -160.3817)
  line L112 (82.3989, -160.3817) -> (82.3989, -149.1552)
  line L113 (85.8146, -149.1552) -> (85.8146, -160.3817)
  line L114 (85.8146, -160.3817) -> (84.6762, -160.3817)
  line L115 (84.6762, -160.3817) -> (84.6762, -149.1552)
  spline S261 degree 3 poles (84.6762, -149.1552) (84.6762, -147.1629) (84.038, -145.5816) (82.7626, -144.4113) knots 0 0 0 0 1 1 1 1
  spline S262 degree 3 poles (82.7626, -144.4113) (81.4872, -143.2311) (79.8482, -142.6407) (77.8454, -142.6407) knots 0 0 0 0 1 1 1 1
  spline S263 degree 3 poles (77.8454, -142.6407) (75.9901, -142.6407) (74.4402, -143.257) (73.1966, -144.4906) knots 0 0 0 0 1 1 1 1
  spline S264 degree 3 poles (73.1966, -144.4906) (71.9526, -145.7241) (71.3304, -147.2262) (71.3304, -148.9968) knots 0 0 0 0 1 1 1 1
  spline S265 degree 3 poles (71.3304, -148.9968) (71.3304, -150.0724) (71.5152, -151.0369) (71.8839, -151.8909) knots 0 0 0 0 1 1 1 1
  spline S266 degree 3 poles (71.8839, -151.8909) (72.2635, -152.7443) (72.7747, -153.4298) (73.4178, -153.9465) knots 0 0 0 0 1 1 1 1
  spline S267 degree 3 poles (73.4178, -153.9465) (74.061, -154.4626) (74.7774, -154.8582) (75.5681, -155.1322) knots 0 0 0 0 1 1 1 1
  spline S268 degree 3 poles (75.5681, -155.1322) (76.3692, -155.3957) (77.2127, -155.5272) (78.098, -155.5272) knots 0 0 0 0 1 1 1 1
  spline S269 degree 3 poles (78.098, -155.5272) (79.3001, -155.5272) (80.4435, -155.2483) (81.5296, -154.6893) knots 0 0 0 0 1 1 1 1
  line L116 (81.5296, -154.6893) -> (81.5296, -155.891)
  spline S270 degree 3 poles (81.5296, -155.891) (80.3907, -156.3652) (79.2418, -156.6029) (78.0825, -156.6029) knots 0 0 0 0 1 1 1 1
  spline S271 degree 3 poles (78.0825, -156.6029) (77.0388, -156.6029) (76.0479, -156.4444) (75.1097, -156.1281) knots 0 0 0 0 1 1 1 1
  spline S272 degree 3 poles (75.1097, -156.1281) (74.1716, -155.8013) (73.3336, -155.3325) (72.5953, -154.7212) knots 0 0 0 0 1 1 1 1
  spline S273 degree 3 poles (72.5953, -154.7212) (71.8575, -154.0989) (71.2726, -153.2978) (70.8406, -152.3173) knots 0 0 0 0 1 1 1 1
  spline S274 degree 3 poles (70.8406, -152.3173) (70.4082, -151.3269) (70.192, -150.2199) (70.192, -148.9968) knots 0 0 0 0 1 1 1 1
  spline S275 degree 3 poles (70.192, -148.9968) (70.192, -146.9203) (70.9248, -145.1547) (72.3901, -143.6999) knots 0 0 0 0 1 1 1 1
  spline S276 degree 3 poles (72.3901, -143.6999) (73.8657, -142.2347) (75.6842, -141.5018) (77.8454, -141.5018) knots 0 0 0 0 1 1 1 1
  spline S277 degree 3 poles (77.8454, -141.5018) (79.3629, -141.5018) (80.723, -141.8132) (81.9247, -142.435) knots 0 0 0 0 1 1 1 1
  spline S278 degree 3 poles (81.9247, -142.435) (83.1263, -143.0463) (84.0749, -143.9371) (84.7709, -145.1073) knots 0 0 0 0 1 1 1 1
  spline S279 degree 3 poles (84.7709, -145.1073) (85.4664, -146.2771) (85.8146, -147.6268) (85.8146, -149.1552) knots 0 0 0 0 1 1 1 1
  line L117 (88.0914, -149.1552) -> (88.0914, -160.3817)
  line L118 (88.0914, -160.3817) -> (86.953, -160.3817)
  line L119 (86.953, -160.3817) -> (86.953, -149.1552)
  spline S280 degree 3 poles (86.953, -149.1552) (86.953, -147.416) (86.5525, -145.8766) (85.7514, -144.5379) knots 0 0 0 0 1 1 1 1
  spline S281 degree 3 poles (85.7514, -144.5379) (84.9607, -143.1888) (83.8746, -142.1555) (82.4941, -141.4391) knots 0 0 0 0 1 1 1 1
  spline S282 degree 3 poles (82.4941, -141.4391) (81.1131, -140.7222) (79.5632, -140.3634) (77.8454, -140.3634) knots 0 0 0 0 1 1 1 1
  spline S283 degree 3 poles (77.8454, -140.3634) (76.2113, -140.3634) (74.7197, -140.7535) (73.3705, -141.5337) knots 0 0 0 0 1 1 1 1
  spline S284 degree 3 poles (73.3705, -141.5337) (72.0209, -142.3035) (70.9617, -143.3467) (70.192, -144.6644) knots 0 0 0 0 1 1 1 1
  spline S285 degree 3 poles (70.192, -144.6644) (69.4332, -145.9822) (69.0536, -147.4265) (69.0536, -148.9968) knots 0 0 0 0 1 1 1 1
  spline S286 degree 3 poles (69.0536, -148.9968) (69.0536, -150.3464) (69.3012, -151.5795) (69.7969, -152.697) knots 0 0 0 0 1 1 1 1
  spline S287 degree 3 poles (69.7969, -152.697) (70.2921, -153.804) (70.9562, -154.7157) (71.7892, -155.4326) knots 0 0 0 0 1 1 1 1
  spline S288 degree 3 poles (71.7892, -155.4326) (72.6327, -156.1495) (73.5862, -156.708) (74.6509, -157.1085) knots 0 0 0 0 1 1 1 1
  spline S289 degree 3 poles (74.6509, -157.1085) (75.7265, -157.4987) (76.849, -157.6934) (78.0192, -157.6934) knots 0 0 0 0 1 1 1 1
  spline S290 degree 3 poles (78.0192, -157.6934) (79.2105, -157.6934) (80.3802, -157.4458) (81.5296, -156.9506) knots 0 0 0 0 1 1 1 1
  line L120 (81.5296, -156.9506) -> (81.5296, -158.105)
  spline S291 degree 3 poles (81.5296, -158.105) (80.3274, -158.5583) (79.1472, -158.7845) (77.9874, -158.7845) knots 0 0 0 0 1 1 1 1
  spline S292 degree 3 poles (77.9874, -158.7845) (76.1639, -158.7845) (74.4875, -158.3735) (72.959, -157.5514) knots 0 0 0 0 1 1 1 1
  spline S293 degree 3 poles (72.959, -157.5514) (71.4305, -156.7289) (70.2079, -155.5641) (69.2907, -154.0571) knots 0 0 0 0 1 1 1 1
  spline S294 degree 3 poles (69.2907, -154.0571) (68.3735, -152.5495) (67.9152, -150.8631) (67.9152, -148.9968) knots 0 0 0 0 1 1 1 1
  spline S295 degree 3 poles (67.9152, -148.9968) (67.9152, -147.6686) (68.1683, -146.4037) (68.674, -145.202) knots 0 0 0 0 1 1 1 1
  spline S296 degree 3 poles (68.674, -145.202) (69.1906, -144.0003) (69.8866, -142.9621) (70.7614, -142.0872) knots 0 0 0 0 1 1 1 1
  spline S297 degree 3 poles (70.7614, -142.0872) (71.6363, -141.2124) (72.6905, -140.5164) (73.9235, -139.9998) knots 0 0 0 0 1 1 1 1
  spline S298 degree 3 poles (73.9235, -139.9998) (75.1571, -139.4836) (76.4644, -139.2251) (77.8454, -139.2251) knots 0 0 0 0 1 1 1 1
  spline S299 degree 3 poles (77.8454, -139.2251) (79.7744, -139.2251) (81.5136, -139.6361) (83.0631, -140.4586) knots 0 0 0 0 1 1 1 1
  spline S300 degree 3 poles (83.0631, -140.4586) (84.6234, -141.2806) (85.8515, -142.4509) (86.7473, -143.969) knots 0 0 0 0 1 1 1 1
  spline S301 degree 3 poles (86.7473, -143.969) (87.6435, -145.487) (88.0914, -147.2157) (88.0914, -149.1552) knots 0 0 0 0 1 1 1 1
  line L121 (90.3682, -149.1552) -> (90.3682, -160.3817)
  line L122 (90.3682, -160.3817) -> (89.2298, -160.3817)
  line L123 (89.2298, -160.3817) -> (89.2298, -149.1552)
  spline S302 degree 3 poles (89.2298, -149.1552) (89.2298, -147.0045) (88.7291, -145.0864) (87.7277, -143.3995) knots 0 0 0 0 1 1 1 1
  spline S303 degree 3 poles (87.7277, -143.3995) (86.7263, -141.7026) (85.3613, -140.3953) (83.6325, -139.4781) knots 0 0 0 0 1 1 1 1
  spline S304 degree 3 poles (83.6325, -139.4781) (81.9037, -138.5505) (79.9747, -138.0867) (77.8454, -138.0867) knots 0 0 0 0 1 1 1 1
  spline S305 degree 3 poles (77.8454, -138.0867) (75.8003, -138.0867) (73.929, -138.5769) (72.2316, -139.5574) knots 0 0 0 0 1 1 1 1
  spline S306 degree 3 poles (72.2316, -139.5574) (70.5347, -140.5373) (69.2011, -141.8655) (68.2316, -143.542) knots 0 0 0 0 1 1 1 1
  spline S307 degree 3 poles (68.2316, -143.542) (67.2616, -145.2075) (66.7768, -147.0259) (66.7768, -148.9968) knots 0 0 0 0 1 1 1 1
  spline S308 degree 3 poles (66.7768, -148.9968) (66.7768, -150.2936) (66.9821, -151.5272) (67.3936, -152.697) knots 0 0 0 0 1 1 1 1
  spline S309 degree 3 poles (67.3936, -152.697) (67.8151, -153.8568) (68.3845, -154.8736) (69.1009, -155.749) knots 0 0 0 0 1 1 1 1
  spline S310 degree 3 poles (69.1009, -155.749) (69.8283, -156.6133) (70.6613, -157.3616) (71.5994, -157.9944) knots 0 0 0 0 1 1 1 1
  spline S311 degree 3 poles (71.5994, -157.9944) (72.548, -158.6266) (73.5653, -159.1063) (74.6509, -159.4332) knots 0 0 0 0 1 1 1 1
  spline S312 degree 3 poles (74.6509, -159.4332) (75.7474, -159.76) (76.8594, -159.9234) (77.9874, -159.9234) knots 0 0 0 0 1 1 1 1
  spline S313 degree 3 poles (77.9874, -159.9234) (79.2314, -159.9234) (80.4121, -159.6863) (81.5296, -159.2115) knots 0 0 0 0 1 1 1 1
  line L124 (81.5296, -159.2115) -> (81.5296, -160.3817)
  spline S314 degree 3 poles (81.5296, -160.3817) (80.3593, -160.7928) (79.1576, -160.9985) (77.9241, -160.9985) knots 0 0 0 0 1 1 1 1
  spline S315 degree 3 poles (77.9241, -160.9985) (76.6487, -160.9985) (75.4047, -160.8192) (74.1925, -160.461) knots 0 0 0 0 1 1 1 1
  spline S316 degree 3 poles (74.1925, -160.461) (72.9909, -160.1023) (71.8734, -159.5751) (70.8406, -158.8797) knots 0 0 0 0 1 1 1 1
  spline S317 degree 3 poles (70.8406, -158.8797) (69.8178, -158.1732) (68.9166, -157.3457) (68.1364, -156.3971) knots 0 0 0 0 1 1 1 1
  spline S318 degree 3 poles (68.1364, -156.3971) (67.3567, -155.4376) (66.7449, -154.3206) (66.3025, -153.0447) knots 0 0 0 0 1 1 1 1
  spline S319 degree 3 poles (66.3025, -153.0447) (65.8596, -151.7693) (65.6384, -150.4202) (65.6384, -148.9968) knots 0 0 0 0 1 1 1 1
  spline S320 degree 3 poles (65.6384, -148.9968) (65.6384, -147.3632) (65.9438, -145.8083) (66.5551, -144.3326) knots 0 0 0 0 1 1 1 1
  spline S321 degree 3 poles (66.5551, -144.3326) (67.1774, -142.846) (68.0208, -141.5651) (69.0855, -140.49) knots 0 0 0 0 1 1 1 1
  spline S322 degree 3 poles (69.0855, -140.49) (70.1606, -139.4044) (71.4569, -138.545) (72.9749, -137.9128) knots 0 0 0 0 1 1 1 1
  spline S323 degree 3 poles (72.9749, -137.9128) (74.5034, -137.2696) (76.1271, -136.9483) (77.8454, -136.9483) knots 0 0 0 0 1 1 1 1
  spline S324 degree 3 poles (77.8454, -136.9483) (79.5951, -136.9483) (81.2396, -137.2432) (82.7786, -137.8336) knots 0 0 0 0 1 1 1 1
  spline S325 degree 3 poles (82.7786, -137.8336) (84.3175, -138.4239) (85.6457, -139.246) (86.7632, -140.3002) knots 0 0 0 0 1 1 1 1
  spline S326 degree 3 poles (86.7632, -140.3002) (87.8807, -141.3439) (88.761, -142.6298) (89.4037, -144.1588) knots 0 0 0 0 1 1 1 1
  spline S327 degree 3 poles (89.4037, -144.1588) (90.0469, -145.6872) (90.3682, -147.3528) (90.3682, -149.1552) knots 0 0 0 0 1 1 1 1
  line L125 (103.6503, -149.5503) -> (101.8478, -149.5503)
  spline S328 degree 3 poles (101.8478, -149.5503) (99.6343, -149.5503) (97.9319, -149.1024) (96.7407, -148.2067) knots 0 0 0 0 1 1 1 1
  spline S329 degree 3 poles (96.7407, -148.2067) (95.5495, -147.2999) (94.9537, -146.0559) (94.9537, -144.4746) knots 0 0 0 0 1 1 1 1
  spline S330 degree 3 poles (94.9537, -144.4746) (94.9537, -142.9989) (95.6546, -141.7709) (97.0571, -140.7904) knots 0 0 0 0 1 1 1 1